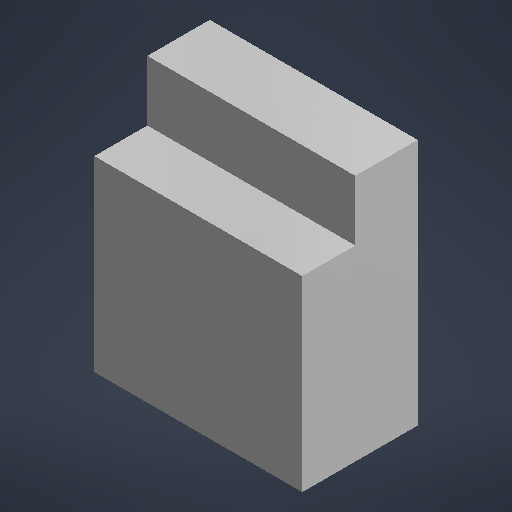
# Autodesk Inventor part: coffretElec
Saved by Autodesk Inventor 2026.2 (Build 302298010, 298A)
## iProperties
Part Number: coffretElec
Material: Générique
Document SubType Name: Modélisation
Designer: quent
Appearance: Par défaut
Author: quent
Autodesk Inventor part; units mm, degrees
ref_plane "Plan YZ" through (0, 0, 0) normal (1, 0, 0) x (0, 1, 0)
ref_plane "Plan XZ" through (0, 0, 0) normal (0, 1, 0) x (-1, 0, 0)
ref_plane "Plan XY" through (0, 0, 0) normal (0, 0, 1) x (1, 0, 0)
sketch "Esquisse1" plane through (0, 0, 0) normal (0, 0, 1) x (1, 0, 0)
  line L0 (0, 0) -> (200, 0)
  line L1 (200, 0) -> (200, 238)
  line L2 (200, 238) -> (0, 238)
  line L3 (0, 238) -> (0, 0)
  line L4 (0, 0) -> (200, 0)
  line L5 (200, 0) -> (200, 180)
  line L6 (200, 180) -> (0, 180)
  line L7 (0, 180) -> (0, 0)
  point P0 (0, 180)
  dimension "d0" = 200
  dimension "d1" = 238
  dimension "d2" = 180
  constraints: 16 end point, 4 parallel, 2 horizontal, 2 perpendicular, 1 point on line
  measures "d0" distance between parallel lines of L3 L1
  measures "d1" distance between parallel lines of L0 L2
  measures "d2" distance between parallel lines of L0 L6
extrude "Extrusion1" add sketch "Esquisse1" along normal blind 111 contours L3 L6 L1 L0
extrude "Extrusion2" add sketch "Esquisse1" along normal blind 60 contours L3 L2 L1 L6
